Autodesk Inventor part; units mm, degrees
(part 2 of 4)
  line L580 (32.3405, 31.3602) -> (32.5714, 31.19) construction
  spline S108 degree 2 poles (32.5714, 31.19) (32.7659, 31.0482) (32.9604, 30.5985) (32.9604, 30.3229) knots 0 0 0 1 2 2 2
  line L581 (32.5714, 31.19) -> (32.7659, 31.0482) construction
  line L582 (32.7659, 31.0482) -> (32.9604, 30.5985) construction
  line L583 (32.9604, 30.5985) -> (32.9604, 30.3229) construction
  spline S109 degree 2 poles (32.9604, 30.3229) (32.9604, 30.0515) (32.7416, 29.6058) (32.5552, 29.468) knots 0 0 0 1 2 2 2
  line L584 (32.9604, 30.3229) -> (32.9604, 30.0515) construction
  line L585 (32.9604, 30.0515) -> (32.7416, 29.6058) construction
  line L586 (32.7416, 29.6058) -> (32.5552, 29.468) construction
  spline S110 degree 2 poles (35.9385, 29.5571) (35.7076, 29.7962) (35.4523, 30.5336) (35.4523, 31.028) knots 0 0 0 1 2 2 2
  line L587 (35.9385, 29.5571) -> (35.7076, 29.7962) construction
  line L588 (35.7076, 29.7962) -> (35.4523, 30.5336) construction
  line L589 (35.4523, 30.5336) -> (35.4523, 31.028) construction
  spline S111 degree 2 poles (35.4523, 31.028) (35.4523, 31.5223) (35.7157, 32.2435) (35.9385, 32.4866) knots 0 0 0 1 2 2 2
  line L590 (35.4523, 31.028) -> (35.4523, 31.5223) construction
  line L591 (35.4523, 31.5223) -> (35.7157, 32.2435) construction
  line L592 (35.7157, 32.2435) -> (35.9385, 32.4866) construction
  spline S112 degree 2 poles (35.9385, 32.4866) (36.1614, 32.7338) (36.8219, 32.9972) (37.2027, 32.9972) knots 0 0 0 1 2 2 2
  line L593 (35.9385, 32.4866) -> (36.1614, 32.7338) construction
  line L594 (36.1614, 32.7338) -> (36.8219, 32.9972) construction
  line L595 (36.8219, 32.9972) -> (37.2027, 32.9972) construction
  spline S113 degree 2 poles (37.2027, 32.9972) (37.5107, 32.9972) (38.086, 32.8229) (38.3089, 32.7095) knots 0 0 0 1 2 2 2
  line L596 (37.2027, 32.9972) -> (37.5107, 32.9972) construction
  line L597 (37.5107, 32.9972) -> (38.086, 32.8229) construction
  line L598 (38.086, 32.8229) -> (38.3089, 32.7095) construction
  spline S114 degree 2 poles (38.2724, 32.0004) (38.2035, 32.0571) (37.9928, 32.203) (37.8429, 32.28) knots 0 0 0 1 2 2 2
  line L599 (38.2724, 32.0004) -> (38.2035, 32.0571) construction
  line L600 (38.2035, 32.0571) -> (37.9928, 32.203) construction
  line L601 (37.9928, 32.203) -> (37.8429, 32.28) construction
  spline S115 degree 2 poles (37.8429, 32.28) (37.7092, 32.3448) (37.3526, 32.4461) (37.1906, 32.4461) knots 0 0 0 1 2 2 2
  line L602 (37.8429, 32.28) -> (37.7092, 32.3448) construction
  line L603 (37.7092, 32.3448) -> (37.3526, 32.4461) construction
  line L604 (37.3526, 32.4461) -> (37.1906, 32.4461) construction
  spline S116 degree 2 poles (37.1906, 32.4461) (36.7003, 32.4461) (36.1047, 31.7046) (36.1047, 31.028) knots 0 0 0 1 2 2 2
  line L605 (37.1906, 32.4461) -> (36.7003, 32.4461) construction
  line L606 (36.7003, 32.4461) -> (36.1047, 31.7046) construction
  line L607 (36.1047, 31.7046) -> (36.1047, 31.028) construction
  spline S117 degree 2 poles (36.1047, 31.028) (36.1047, 30.3675) (36.68, 29.626) (37.1906, 29.626) knots 0 0 0 1 2 2 2
  line L608 (36.1047, 31.028) -> (36.1047, 30.3675) construction
  line L609 (36.1047, 30.3675) -> (36.68, 29.626) construction
  line L610 (36.68, 29.626) -> (37.1906, 29.626) construction
  spline S118 degree 2 poles (37.1906, 29.626) (37.4985, 29.626) (38.0577, 29.8813) (38.2724, 30.0798) knots 0 0 0 1 2 2 2
  line L611 (37.1906, 29.626) -> (37.4985, 29.626) construction
  line L612 (37.4985, 29.626) -> (38.0577, 29.8813) construction
  line L613 (38.0577, 29.8813) -> (38.2724, 30.0798) construction
  spline S119 degree 2 poles (38.3089, 29.3707) (38.2157, 29.3262) (37.9321, 29.2006) (37.8186, 29.1722) knots 0 0 0 1 2 2 2
  line L614 (38.3089, 29.3707) -> (38.2157, 29.3262) construction
  line L615 (38.2157, 29.3262) -> (37.9321, 29.2006) construction
  line L616 (37.9321, 29.2006) -> (37.8186, 29.1722) construction
  spline S120 degree 2 poles (37.8186, 29.1722) (37.6565, 29.1236) (37.4013, 29.075) (37.2027, 29.075) knots 0 0 0 1 2 2 2
  line L617 (37.8186, 29.1722) -> (37.6565, 29.1236) construction
  line L618 (37.6565, 29.1236) -> (37.4013, 29.075) construction
  line L619 (37.4013, 29.075) -> (37.2027, 29.075) construction
  spline S121 degree 2 poles (37.2027, 29.075) (36.8138, 29.075) (36.1695, 29.314) (35.9385, 29.5571) knots 0 0 0 1 2 2 2
  line L620 (37.2027, 29.075) -> (36.8138, 29.075) construction
  line L621 (36.8138, 29.075) -> (36.1695, 29.314) construction
  line L622 (36.1695, 29.314) -> (35.9385, 29.5571) construction
  spline S122 degree 2 poles (36.6071, 21.7178) (36.4937, 21.4504) (36.21, 21.1303) (36.0561, 21.0492) knots 0 0 0 1 2 2 2
  line L623 (36.6071, 21.7178) -> (36.4937, 21.4504) construction
  line L624 (36.4937, 21.4504) -> (36.21, 21.1303) construction
  line L625 (36.21, 21.1303) -> (36.0561, 21.0492) construction
  spline S123 degree 2 poles (36.0561, 21.0492) (35.898, 20.9641) (35.6022, 20.9115) (35.4483, 20.9115) knots 0 0 0 1 2 2 2
  line L626 (36.0561, 21.0492) -> (35.898, 20.9641) construction
  line L627 (35.898, 20.9641) -> (35.6022, 20.9115) construction
  line L628 (35.6022, 20.9115) -> (35.4483, 20.9115) construction
  spline S124 degree 2 poles (35.4483, 20.9115) (35.3146, 20.9115) (34.9499, 20.9236) (34.9013, 20.9277) knots 0 0 0 1 2 2 2
  line L629 (35.4483, 20.9115) -> (35.3146, 20.9115) construction
  line L630 (35.3146, 20.9115) -> (34.9499, 20.9236) construction
  line L631 (34.9499, 20.9236) -> (34.9013, 20.9277) construction
  spline S125 degree 2 poles (34.9499, 21.5517) (34.9985, 21.5436) (35.2052, 21.5274) (35.3632, 21.5274) knots 0 0 0 1 2 2 2
  line L632 (34.9499, 21.5517) -> (34.9985, 21.5436) construction
  line L633 (34.9985, 21.5436) -> (35.2052, 21.5274) construction
  line L634 (35.2052, 21.5274) -> (35.3632, 21.5274) construction
  spline S126 degree 2 poles (35.3632, 21.5274) (35.4361, 21.5274) (35.6387, 21.5436) (35.7238, 21.5841) knots 0 0 0 1 2 2 2
  line L635 (35.3632, 21.5274) -> (35.4361, 21.5274) construction
  line L636 (35.4361, 21.5274) -> (35.6387, 21.5436) construction
  line L637 (35.6387, 21.5436) -> (35.7238, 21.5841) construction
  spline S127 degree 2 poles (35.7238, 21.5841) (35.821, 21.6327) (35.9912, 21.7867) (36.0601, 21.9609) knots 0 0 0 1 2 2 2
  line L638 (35.7238, 21.5841) -> (35.821, 21.6327) construction
  line L639 (35.821, 21.6327) -> (35.9912, 21.7867) construction
  line L640 (35.9912, 21.7867) -> (36.0601, 21.9609) construction
  spline S128 degree 2 poles (23.4711, -2.5288) (23.0697, -2.5288) (22.4735, -1.952) (22.4735, -1.5311) knots 0 0 0 1 2 2 2
  line L641 (23.4711, -2.5288) -> (23.0697, -2.5288) construction
  line L642 (23.0697, -2.5288) -> (22.4735, -1.952) construction
  line L643 (22.4735, -1.952) -> (22.4735, -1.5311) construction
  line L644 (22.4735, -1.5311) -> (22.4735, -0.0346)
  spline S129 degree 2 poles (22.4735, -0.0346) (22.4735, 0.3785) (23.058, 0.963) (23.4711, 0.963) knots 0 0 0 1 2 2 2
  line L645 (22.4735, -0.0346) -> (22.4735, 0.3785) construction
  line L646 (22.4735, 0.3785) -> (23.058, 0.963) construction
  line L647 (23.058, 0.963) -> (23.4711, 0.963) construction
  line L648 (23.4711, 0.963) -> (24.2194, 0.963)
  spline S130 degree 2 poles (24.2194, 0.963) (24.3207, 0.963) (24.4688, 0.8111) (24.4688, 0.7136) knots 0 0 0 1 2 2 2
  line L649 (24.2194, 0.963) -> (24.3207, 0.963) construction
  line L650 (24.3207, 0.963) -> (24.4688, 0.8111) construction
  line L651 (24.4688, 0.8111) -> (24.4688, 0.7136) construction
  spline S131 degree 2 poles (24.4688, 0.7136) (24.4688, 0.6279) (24.3441, 0.4642) (24.2194, 0.4642) knots 0 0 0 1 2 2 2
  line L652 (24.4688, 0.7136) -> (24.4688, 0.6279) construction
  line L653 (24.4688, 0.6279) -> (24.3441, 0.4642) construction
  line L654 (24.3441, 0.4642) -> (24.2194, 0.4642) construction
  line L655 (24.2194, 0.4642) -> (23.4711, 0.4642)
  spline S132 degree 2 poles (23.4711, 0.4642) (23.2607, 0.4642) (23.1165, 0.32) knots 0 0 0 1 1 1
  line L656 (23.4711, 0.4642) -> (23.2607, 0.4642) construction
  line L657 (23.2607, 0.4642) -> (23.1165, 0.32) construction
  spline S133 degree 2 poles (23.1165, 0.32) (23.0424, 0.2499) (22.9723, 0.0706) (22.9723, -0.0346) knots 0 0 0 1 2 2 2
  line L658 (23.1165, 0.32) -> (23.0424, 0.2499) construction
  line L659 (23.0424, 0.2499) -> (22.9723, 0.0706) construction
  line L660 (22.9723, 0.0706) -> (22.9723, -0.0346) construction
  line L661 (22.9723, -0.0346) -> (22.9723, -1.5311)
  spline S134 degree 2 poles (22.9723, -1.5311) (22.9723, -1.7415) (23.1165, -1.8857) knots 0 0 0 1 1 1
  line L662 (22.9723, -1.5311) -> (22.9723, -1.7415) construction
  line L663 (22.9723, -1.7415) -> (23.1165, -1.8857) construction
  spline S135 degree 2 poles (23.1165, -1.8857) (23.1905, -1.952) (23.2763, -1.9949) knots 0 0 0 1 1 1
  line L664 (23.1165, -1.8857) -> (23.1905, -1.952) construction
  line L665 (23.1905, -1.952) -> (23.2763, -1.9949) construction
  spline S136 degree 2 poles (23.2763, -1.9949) (23.3815, -2.0299) (23.4711, -2.0299) knots 0 0 0 1 1 1
  line L666 (23.2763, -1.9949) -> (23.3815, -2.0299) construction
  line L667 (23.3815, -2.0299) -> (23.4711, -2.0299) construction
  line L668 (23.4711, -2.0299) -> (24.2194, -2.0299)
  spline S137 degree 2 poles (24.2194, -2.0299) (24.3207, -2.0299) (24.4688, -2.1819) (24.4688, -2.2794) knots 0 0 0 1 2 2 2
  line L669 (24.2194, -2.0299) -> (24.3207, -2.0299) construction
  line L670 (24.3207, -2.0299) -> (24.4688, -2.1819) construction
  line L671 (24.4688, -2.1819) -> (24.4688, -2.2794) construction
  spline S138 degree 2 poles (24.4688, -2.2794) (24.4688, -2.3651) (24.3441, -2.5288) (24.2194, -2.5288) knots 0 0 0 1 2 2 2
  line L672 (24.4688, -2.2794) -> (24.4688, -2.3651) construction
  line L673 (24.4688, -2.3651) -> (24.3441, -2.5288) construction
  line L674 (24.3441, -2.5288) -> (24.2194, -2.5288) construction
  line L675 (24.2194, -2.5288) -> (23.4711, -2.5288)
  spline S139 degree 2 poles (2.1309, -41.5414) (1.6445, -41.5414) (0.9337, -40.8446) (0.9337, -40.3442) knots 0 0 0 1 2 2 2
  line L676 (2.1309, -41.5414) -> (1.6445, -41.5414) construction
  line L677 (1.6445, -41.5414) -> (0.9337, -40.8446) construction
  line L678 (0.9337, -40.8446) -> (0.9337, -40.3442) construction
  line L679 (0.9337, -40.3442) -> (0.9337, -36.7526)
  spline S140 degree 2 poles (0.9337, -36.7526) (0.9337, -36.2522) (1.6305, -35.5554) (2.1309, -35.5554) knots 0 0 0 1 2 2 2
  line L680 (0.9337, -36.7526) -> (0.9337, -36.2522) construction
  line L681 (0.9337, -36.2522) -> (1.6305, -35.5554) construction
  line L682 (1.6305, -35.5554) -> (2.1309, -35.5554) construction
  line L683 (2.1309, -35.5554) -> (3.6274, -35.5554)
  spline S141 degree 2 poles (3.6274, -35.5554) (3.749, -35.5554) (3.9267, -35.7378) (3.9267, -35.8547) knots 0 0 0 1 2 2 2
  line L684 (3.6274, -35.5554) -> (3.749, -35.5554) construction
  line L685 (3.749, -35.5554) -> (3.9267, -35.7378) construction
  line L686 (3.9267, -35.7378) -> (3.9267, -35.8547) construction
  spline S142 degree 2 poles (3.9267, -35.8547) (3.9267, -35.9576) (3.777, -36.154) (3.6274, -36.154) knots 0 0 0 1 2 2 2
  line L687 (3.9267, -35.8547) -> (3.9267, -35.9576) construction
  line L688 (3.9267, -35.9576) -> (3.777, -36.154) construction
  line L689 (3.777, -36.154) -> (3.6274, -36.154) construction
  line L690 (3.6274, -36.154) -> (2.1309, -36.154)
  spline S143 degree 2 poles (2.1309, -36.154) (1.8784, -36.154) (1.7053, -36.3271) knots 0 0 0 1 1 1
  line L691 (2.1309, -36.154) -> (1.8784, -36.154) construction
  line L692 (1.8784, -36.154) -> (1.7053, -36.3271) construction
  spline S144 degree 2 poles (1.7053, -36.3271) (1.6165, -36.4112) (1.5323, -36.6263) (1.5323, -36.7526) knots 0 0 0 1 2 2 2
  line L693 (1.7053, -36.3271) -> (1.6165, -36.4112) construction
  line L694 (1.6165, -36.4112) -> (1.5323, -36.6263) construction
  line L695 (1.5323, -36.6263) -> (1.5323, -36.7526) construction
  line L696 (1.5323, -36.7526) -> (1.5323, -40.3442)
  spline S145 degree 2 poles (1.5323, -40.3442) (1.5323, -40.5967) (1.7053, -40.7698) knots 0 0 0 1 1 1
  line L697 (1.5323, -40.3442) -> (1.5323, -40.5967) construction
  line L698 (1.5323, -40.5967) -> (1.7053, -40.7698) construction
  spline S146 degree 2 poles (1.7053, -40.7698) (1.7942, -40.8493) (1.8971, -40.9007) knots 0 0 0 1 1 1
  line L699 (1.7053, -40.7698) -> (1.7942, -40.8493) construction
  line L700 (1.7942, -40.8493) -> (1.8971, -40.9007) construction
  spline S147 degree 2 poles (1.8971, -40.9007) (2.0233, -40.9428) (2.1309, -40.9428) knots 0 0 0 1 1 1
  line L701 (1.8971, -40.9007) -> (2.0233, -40.9428) construction
  line L702 (2.0233, -40.9428) -> (2.1309, -40.9428) construction
  line L703 (2.1309, -40.9428) -> (3.6274, -40.9428)
  spline S148 degree 2 poles (3.6274, -40.9428) (3.749, -40.9428) (3.9267, -41.1252) (3.9267, -41.2421) knots 0 0 0 1 2 2 2
  line L704 (3.6274, -40.9428) -> (3.749, -40.9428) construction
  line L705 (3.749, -40.9428) -> (3.9267, -41.1252) construction
  line L706 (3.9267, -41.1252) -> (3.9267, -41.2421) construction
  spline S149 degree 2 poles (3.9267, -41.2421) (3.9267, -41.345) (3.777, -41.5414) (3.6274, -41.5414) knots 0 0 0 1 2 2 2
  line L707 (3.9267, -41.2421) -> (3.9267, -41.345) construction
  line L708 (3.9267, -41.345) -> (3.777, -41.5414) construction
  line L709 (3.777, -41.5414) -> (3.6274, -41.5414) construction
  line L710 (3.6274, -41.5414) -> (2.1309, -41.5414)
  spline S150 degree 2 poles (-5.1364, -41.4666) (-5.2206, -41.5414) (-5.3516, -41.5414) knots 0 0 0 1 1 1
  line L711 (-5.1364, -41.4666) -> (-5.2206, -41.5414) construction
  line L712 (-5.2206, -41.5414) -> (-5.3516, -41.5414) construction
  spline S151 degree 2 poles (-5.3516, -41.5414) (-5.4732, -41.5414) (-5.6509, -41.3917) (-5.6509, -41.2421) knots 0 0 0 1 2 2 2
  line L713 (-5.3516, -41.5414) -> (-5.4732, -41.5414) construction
  line L714 (-5.4732, -41.5414) -> (-5.6509, -41.3917) construction
  line L715 (-5.6509, -41.3917) -> (-5.6509, -41.2421) construction
  spline S152 degree 2 poles (-8.0452, -41.2421) (-8.0452, -41.3824) (-8.1294, -41.4666) knots 0 0 0 1 1 1
  line L716 (-8.0452, -41.2421) -> (-8.0452, -41.3824) construction
  line L717 (-8.0452, -41.3824) -> (-8.1294, -41.4666) construction
  spline S153 degree 2 poles (-8.1294, -41.4666) (-8.2136, -41.5414) (-8.3445, -41.5414) knots 0 0 0 1 1 1
  line L718 (-8.1294, -41.4666) -> (-8.2136, -41.5414) construction
  line L719 (-8.2136, -41.5414) -> (-8.3445, -41.5414) construction
  spline S154 degree 2 poles (-8.3445, -41.5414) (-8.4661, -41.5414) (-8.6438, -41.3917) (-8.6438, -41.2421) knots 0 0 0 1 2 2 2
  line L720 (-8.3445, -41.5414) -> (-8.4661, -41.5414) construction
  line L721 (-8.4661, -41.5414) -> (-8.6438, -41.3917) construction
  line L722 (-8.6438, -41.3917) -> (-8.6438, -41.2421) construction
  line L723 (-8.6438, -41.2421) -> (-8.6438, -35.8547)
  spline S155 degree 2 poles (-8.6438, -35.8547) (-8.6438, -35.5554) (-8.3445, -35.5554) knots 0 0 0 1 1 1
  line L724 (-8.6438, -35.8547) -> (-8.6438, -35.5554) construction
  line L725 (-8.6438, -35.5554) -> (-8.3445, -35.5554) construction
  line L726 (-8.3445, -35.5554) -> (-5.3516, -35.5554)
  spline S156 degree 2 poles (-5.3516, -35.5554) (-5.0523, -35.5554) (-5.0523, -35.8547) knots 0 0 0 1 1 1
  line L727 (-5.3516, -35.5554) -> (-5.0523, -35.5554) construction
  line L728 (-5.0523, -35.5554) -> (-5.0523, -35.8547) construction
  line L729 (-5.0523, -35.8547) -> (-5.0523, -41.2421)
  spline S157 degree 2 poles (-5.0523, -41.2421) (-5.0523, -41.3824) (-5.1364, -41.4666) knots 0 0 0 1 1 1
  line L730 (-5.0523, -41.2421) -> (-5.0523, -41.3824) construction
  line L731 (-5.0523, -41.3824) -> (-5.1364, -41.4666) construction
  spline S158 degree 2 poles (-28.9828, -2.8867) (-29.3881, -2.8867) (-29.9804, -2.306) (-29.9804, -1.889) knots 0 0 0 1 2 2 2
  line L732 (-28.9828, -2.8867) -> (-29.3881, -2.8867) construction
  line L733 (-29.3881, -2.8867) -> (-29.9804, -2.306) construction
  line L734 (-29.9804, -2.306) -> (-29.9804, -1.889) construction
  line L735 (-29.9804, -1.889) -> (-29.9804, 1.104)
  spline S159 degree 2 poles (-29.9804, 1.104) (-29.9804, 1.5209) (-29.3998, 2.1016) (-28.9828, 2.1016) knots 0 0 0 1 2 2 2
  line L736 (-29.9804, 1.104) -> (-29.9804, 1.5209) construction
  line L737 (-29.9804, 1.5209) -> (-29.3998, 2.1016) construction
  line L738 (-29.3998, 2.1016) -> (-28.9828, 2.1016) construction
  line L739 (-28.9828, 2.1016) -> (-27.7357, 2.1016)
  spline S160 degree 2 poles (-27.7357, 2.1016) (-27.6344, 2.1016) (-27.4863, 1.9496) (-27.4863, 1.8522) knots 0 0 0 1 2 2 2
  line L740 (-27.7357, 2.1016) -> (-27.6344, 2.1016) construction
  line L741 (-27.6344, 2.1016) -> (-27.4863, 1.9496) construction
  line L742 (-27.4863, 1.9496) -> (-27.4863, 1.8522) construction
  spline S161 degree 2 poles (-27.4863, 1.8522) (-27.4863, 1.7665) (-27.611, 1.6028) (-27.7357, 1.6028) knots 0 0 0 1 2 2 2
  line L743 (-27.4863, 1.8522) -> (-27.4863, 1.7665) construction
  line L744 (-27.4863, 1.7665) -> (-27.611, 1.6028) construction
  line L745 (-27.611, 1.6028) -> (-27.7357, 1.6028) construction
  line L746 (-27.7357, 1.6028) -> (-28.9828, 1.6028)
  spline S162 degree 2 poles (-28.9828, 1.6028) (-29.1932, 1.6028) (-29.3374, 1.4586) knots 0 0 0 1 1 1
  line L747 (-28.9828, 1.6028) -> (-29.1932, 1.6028) construction
  line L748 (-29.1932, 1.6028) -> (-29.3374, 1.4586) construction
  spline S163 degree 2 poles (-29.3374, 1.4586) (-29.4114, 1.3884) (-29.4816, 1.2092) (-29.4816, 1.104) knots 0 0 0 1 2 2 2
  line L749 (-29.3374, 1.4586) -> (-29.4114, 1.3884) construction
  line L750 (-29.4114, 1.3884) -> (-29.4816, 1.2092) construction
  line L751 (-29.4816, 1.2092) -> (-29.4816, 1.104) construction
  line L752 (-29.4816, 1.104) -> (-29.4816, -1.889)
  spline S164 degree 2 poles (-29.4816, -1.889) (-29.4816, -2.0995) (-29.3374, -2.2437) knots 0 0 0 1 1 1
  line L753 (-29.4816, -1.889) -> (-29.4816, -2.0995) construction
  line L754 (-29.4816, -2.0995) -> (-29.3374, -2.2437) construction
  spline S165 degree 2 poles (-29.3374, -2.2437) (-29.2634, -2.3099) (-29.1776, -2.3528) knots 0 0 0 1 1 1
  line L755 (-29.3374, -2.2437) -> (-29.2634, -2.3099) construction
  line L756 (-29.2634, -2.3099) -> (-29.1776, -2.3528) construction
  spline S166 degree 2 poles (-29.1776, -2.3528) (-29.0724, -2.3879) (-28.9828, -2.3879) knots 0 0 0 1 1 1
  line L757 (-29.1776, -2.3528) -> (-29.0724, -2.3879) construction
  line L758 (-29.0724, -2.3879) -> (-28.9828, -2.3879) construction
  line L759 (-28.9828, -2.3879) -> (-27.7357, -2.3879)
  spline S167 degree 2 poles (-27.7357, -2.3879) (-27.6344, -2.3879) (-27.4863, -2.5398) (-27.4863, -2.6373) knots 0 0 0 1 2 2 2
  line L760 (-27.7357, -2.3879) -> (-27.6344, -2.3879) construction
  line L761 (-27.6344, -2.3879) -> (-27.4863, -2.5398) construction
  line L762 (-27.4863, -2.5398) -> (-27.4863, -2.6373) construction
  spline S168 degree 2 poles (-27.4863, -2.6373) (-27.4863, -2.723) (-27.611, -2.8867) (-27.7357, -2.8867) knots 0 0 0 1 2 2 2
  line L763 (-27.4863, -2.6373) -> (-27.4863, -2.723) construction
  line L764 (-27.4863, -2.723) -> (-27.611, -2.8867) construction
  line L765 (-27.611, -2.8867) -> (-27.7357, -2.8867) construction
  line L766 (-27.7357, -2.8867) -> (-28.9828, -2.8867)
  spline S169 degree 2 poles (-36.2158, -0.3964) (-36.3288, -0.3964) (-36.4029, -0.3263) knots 0 0 0 1 1 1
  line L767 (-36.2158, -0.3964) -> (-36.3288, -0.3964) construction
  line L768 (-36.3288, -0.3964) -> (-36.4029, -0.3263) construction
  spline S170 degree 2 poles (-36.4029, -0.3263) (-36.4652, -0.2522) (-36.4652, -0.147) knots 0 0 0 1 1 1
  line L769 (-36.4029, -0.3263) -> (-36.4652, -0.2522) construction
  line L770 (-36.4652, -0.2522) -> (-36.4652, -0.147) construction
  spline S171 degree 2 poles (-36.4652, -0.147) (-36.4652, -0.0574) (-36.3327, 0.1024) (-36.2158, 0.1024) knots 0 0 0 1 2 2 2
  line L771 (-36.4652, -0.147) -> (-36.4652, -0.0574) construction
  line L772 (-36.4652, -0.0574) -> (-36.3327, 0.1024) construction
  line L773 (-36.3327, 0.1024) -> (-36.2158, 0.1024) construction
  spline S172 degree 2 poles (-34.9687, 1.104) (-34.9687, 1.3144) (-35.2493, 1.6028) (-35.4676, 1.6028) knots 0 0 0 1 2 2 2
  line L774 (-34.9687, 1.104) -> (-34.9687, 1.3144) construction
  line L775 (-34.9687, 1.3144) -> (-35.2493, 1.6028) construction
  line L776 (-35.2493, 1.6028) -> (-35.4676, 1.6028) construction
  line L777 (-35.4676, 1.6028) -> (-37.2135, 1.6028)
  spline S173 degree 2 poles (-37.2135, 1.6028) (-37.3265, 1.6028) (-37.4005, 1.669) knots 0 0 0 1 1 1
  line L778 (-37.2135, 1.6028) -> (-37.3265, 1.6028) construction
  line L779 (-37.3265, 1.6028) -> (-37.4005, 1.669) construction
  spline S174 degree 2 poles (-37.4005, 1.669) (-37.4629, 1.7509) (-37.4629, 1.8522) knots 0 0 0 1 1 1
  line L780 (-37.4005, 1.669) -> (-37.4629, 1.7509) construction
  line L781 (-37.4629, 1.7509) -> (-37.4629, 1.8522) construction
  spline S175 degree 2 poles (-37.4629, 1.8522) (-37.4629, 1.9379) (-37.3382, 2.1016) (-37.2135, 2.1016) knots 0 0 0 1 2 2 2
  line L782 (-37.4629, 1.8522) -> (-37.4629, 1.9379) construction
  line L783 (-37.4629, 1.9379) -> (-37.3382, 2.1016) construction
  line L784 (-37.3382, 2.1016) -> (-37.2135, 2.1016) construction
  line L785 (-37.2135, 2.1016) -> (-35.4676, 2.1016)
  spline S176 degree 2 poles (-35.4676, 2.1016) (-35.0506, 2.1016) (-34.4699, 1.517) (-34.4699, 1.104) knots 0 0 0 1 2 2 2
  line L786 (-35.4676, 2.1016) -> (-35.0506, 2.1016) construction
  line L787 (-35.0506, 2.1016) -> (-34.4699, 1.517) construction
  line L788 (-34.4699, 1.517) -> (-34.4699, 1.104) construction
  line L789 (-34.4699, 1.104) -> (-34.4699, -1.889)
  spline S177 degree 2 poles (-34.4699, -1.889) (-34.4699, -2.2982) (-35.0545, -2.8867) (-35.4676, -2.8867) knots 0 0 0 1 2 2 2
  line L790 (-34.4699, -1.889) -> (-34.4699, -2.2982) construction
  line L791 (-34.4699, -2.2982) -> (-35.0545, -2.8867) construction
  line L792 (-35.0545, -2.8867) -> (-35.4676, -2.8867) construction
  line L793 (-35.4676, -2.8867) -> (-37.2135, -2.8867)
  spline S178 degree 2 poles (-37.2135, -2.8867) (-37.3265, -2.8867) (-37.4005, -2.8165) knots 0 0 0 1 1 1
  line L794 (-37.2135, -2.8867) -> (-37.3265, -2.8867) construction
  line L795 (-37.3265, -2.8867) -> (-37.4005, -2.8165) construction
  spline S179 degree 2 poles (-37.4005, -2.8165) (-37.4629, -2.7425) (-37.4629, -2.6373) knots 0 0 0 1 1 1
  line L796 (-37.4005, -2.8165) -> (-37.4629, -2.7425) construction
  line L797 (-37.4629, -2.7425) -> (-37.4629, -2.6373) construction
  spline S180 degree 2 poles (-37.4629, -2.6373) (-37.4629, -2.5476) (-37.3304, -2.3879) (-37.2135, -2.3879) knots 0 0 0 1 2 2 2
  line L798 (-37.4629, -2.6373) -> (-37.4629, -2.5476) construction
  line L799 (-37.4629, -2.5476) -> (-37.3304, -2.3879) construction
  line L800 (-37.3304, -2.3879) -> (-37.2135, -2.3879) construction
  line L801 (-37.2135, -2.3879) -> (-35.4676, -2.3879)
  spline S181 degree 2 poles (-35.4676, -2.3879) (-35.261, -2.3879) (-34.9687, -2.1112) (-34.9687, -1.889) knots 0 0 0 1 2 2 2
  line L802 (-35.4676, -2.3879) -> (-35.261, -2.3879) construction
  line L803 (-35.261, -2.3879) -> (-34.9687, -2.1112) construction
  line L804 (-34.9687, -2.1112) -> (-34.9687, -1.889) construction
  spline S182 degree 2 poles (-26.032, -101.232) (-25.6557, -101.232) (-25.4359, -101.4818) knots 0 0 0 1 1 1
  line L805 (-26.032, -101.232) -> (-25.6557, -101.232) construction
  line L806 (-25.6557, -101.232) -> (-25.4359, -101.4818) construction
  spline S183 degree 2 poles (-25.4359, -101.4818) (-25.236, -101.705) (-25.236, -102.0281) knots 0 0 0 1 1 1
  line L807 (-25.4359, -101.4818) -> (-25.236, -101.705) construction
  line L808 (-25.236, -101.705) -> (-25.236, -102.0281) construction
  spline S184 degree 2 poles (-25.236, -102.0281) (-25.236, -102.3511) (-25.4359, -102.5809) knots 0 0 0 1 1 1
  line L809 (-25.236, -102.0281) -> (-25.236, -102.3511) construction
  line L810 (-25.236, -102.3511) -> (-25.4359, -102.5809) construction
  spline S185 degree 2 poles (-25.4359, -102.5809) (-25.6557, -102.8274) (-26.032, -102.8274) knots 0 0 0 1 1 1
  line L811 (-25.4359, -102.5809) -> (-25.6557, -102.8274) construction
  line L812 (-25.6557, -102.8274) -> (-26.032, -102.8274) construction
  line L813 (-26.032, -102.8274) -> (-26.6315, -102.8274)
  spline S186 degree 2 poles (-26.6315, -102.8274) (-26.8314, -102.8274) (-26.8314, -102.6276) knots 0 0 0 1 1 1
  line L814 (-26.6315, -102.8274) -> (-26.8314, -102.8274) construction
  line L815 (-26.8314, -102.8274) -> (-26.8314, -102.6276) construction
  line L816 (-26.8314, -102.6276) -> (-26.8314, -100.2362)
  spline S187 degree 2 poles (-26.8314, -100.2362) (-26.8314, -100.0364) (-26.6315, -100.0364) knots 0 0 0 1 1 1
  line L817 (-26.8314, -100.2362) -> (-26.8314, -100.0364) construction
  line L818 (-26.8314, -100.0364) -> (-26.6315, -100.0364) construction
  spline S188 degree 2 poles (-26.6315, -100.0364) (-26.4317, -100.0364) (-26.4317, -100.2362) knots 0 0 0 1 1 1
  line L819 (-26.6315, -100.0364) -> (-26.4317, -100.0364) construction
  line L820 (-26.4317, -100.0364) -> (-26.4317, -100.2362) construction
  spline S189 degree 2 poles (-29.2227, -103.8232) (-29.2227, -104.0231) (-29.4225, -104.0231) knots 0 0 0 1 1 1
  line L821 (-29.2227, -103.8232) -> (-29.2227, -104.0231) construction
  line L822 (-29.2227, -104.0231) -> (-29.4225, -104.0231) construction
  spline S190 degree 2 poles (-29.4225, -104.0231) (-29.6224, -104.0231) (-29.6224, -103.8232) knots 0 0 0 1 1 1
  line L823 (-29.4225, -104.0231) -> (-29.6224, -104.0231) construction
  line L824 (-29.6224, -104.0231) -> (-29.6224, -103.8232) construction
  line L825 (-29.6224, -103.8232) -> (-29.6224, -100.2362)
  spline S191 degree 2 poles (-29.6224, -100.2362) (-29.6224, -100.0364) (-29.4225, -100.0364) knots 0 0 0 1 1 1
  line L826 (-29.6224, -100.2362) -> (-29.6224, -100.0364) construction
  line L827 (-29.6224, -100.0364) -> (-29.4225, -100.0364) construction
  line L828 (-29.4225, -100.0364) -> (-28.4267, -100.0364)
  spline S192 degree 2 poles (-28.4267, -100.0364) (-28.097, -100.0364) (-27.6307, -100.5027) (-27.6307, -100.8324) knots 0 0 0 1 2 2 2
  line L829 (-28.4267, -100.0364) -> (-28.097, -100.0364) construction
  line L830 (-28.097, -100.0364) -> (-27.6307, -100.5027) construction
  line L831 (-27.6307, -100.5027) -> (-27.6307, -100.8324) construction
  line L832 (-27.6307, -100.8324) -> (-27.6307, -102.0314)
  spline S193 degree 2 poles (-27.6307, -102.0314) (-27.6307, -102.3611) (-28.097, -102.8274) (-28.4267, -102.8274) knots 0 0 0 1 2 2 2
  line L833 (-27.6307, -102.0314) -> (-27.6307, -102.3611) construction
  line L834 (-27.6307, -102.3611) -> (-28.097, -102.8274) construction
  line L835 (-28.097, -102.8274) -> (-28.4267, -102.8274) construction
  spline S194 degree 2 poles (3.5401, 27.5031) (3.5401, 27.3862) (3.4699, 27.316) knots 0 0 0 1 1 1
  line L836 (3.5401, 27.5031) -> (3.5401, 27.3862) construction
  line L837 (3.5401, 27.3862) -> (3.4699, 27.316) construction
  spline S195 degree 2 poles (3.4699, 27.316) (3.3998, 27.2537) (3.2907, 27.2537) knots 0 0 0 1 1 1
  line L838 (3.4699, 27.316) -> (3.3998, 27.2537) construction
  line L839 (3.3998, 27.2537) -> (3.2907, 27.2537) construction
  spline S196 degree 2 poles (3.2907, 27.2537) (3.1893, 27.2537) (3.0412, 27.3784) (3.0412, 27.5031) knots 0 0 0 1 2 2 2
  line L840 (3.2907, 27.2537) -> (3.1893, 27.2537) construction
  line L841 (3.1893, 27.2537) -> (3.0412, 27.3784) construction
  line L842 (3.0412, 27.3784) -> (3.0412, 27.5031) construction
  line L843 (3.0412, 27.5031) -> (3.0412, 30.4961)
  spline S197 degree 2 poles (3.0412, 30.4961) (3.0412, 30.5935) (3.1153, 30.6793) knots 0 0 0 1 1 1
  line L844 (3.0412, 30.4961) -> (3.0412, 30.5935) construction
  line L845 (3.0412, 30.5935) -> (3.1153, 30.6793) construction
  spline S198 degree 2 poles (3.1153, 30.6793) (3.1893, 30.7455) (3.2907, 30.7455) knots 0 0 0 1 1 1
  line L846 (3.1153, 30.6793) -> (3.1893, 30.7455) construction
  line L847 (3.1893, 30.7455) -> (3.2907, 30.7455) construction
  spline S199 degree 2 poles (3.2907, 30.7455) (3.3881, 30.7455) (3.5401, 30.6208) (3.5401, 30.4961) knots 0 0 0 1 2 2 2
  line L848 (3.2907, 30.7455) -> (3.3881, 30.7455) construction
  line L849 (3.3881, 30.7455) -> (3.5401, 30.6208) construction
  line L850 (3.5401, 30.6208) -> (3.5401, 30.4961) construction
  spline S200 degree 2 poles (5.1223, 30.6831) (5.1847, 30.7572) (5.2821, 30.7572) knots 0 0 0 1 1 1
  line L851 (5.1223, 30.6831) -> (5.1847, 30.7572) construction
  line L852 (5.1847, 30.7572) -> (5.2821, 30.7572) construction
  spline S201 degree 2 poles (5.2821, 30.7572) (5.36, 30.7572) (5.4574, 30.6831) knots 0 0 0 1 1 1
  line L853 (5.2821, 30.7572) -> (5.36, 30.7572) construction
  line L854 (5.36, 30.7572) -> (5.4574, 30.6831) construction
  spline S202 degree 2 poles (5.4574, 30.6831) (5.5315, 30.6091) (5.5315, 30.4922) knots 0 0 0 1 1 1
  line L855 (5.4574, 30.6831) -> (5.5315, 30.6091) construction
  line L856 (5.5315, 30.6091) -> (5.5315, 30.4922) construction
  spline S203 degree 2 poles (5.5315, 30.4922) (5.5315, 30.3909) (5.4497, 30.3051) knots 0 0 0 1 1 1
  line L857 (5.5315, 30.4922) -> (5.5315, 30.3909) construction
  line L858 (5.5315, 30.3909) -> (5.4497, 30.3051) construction
  spline S204 degree 2 poles (5.473, 27.6629) (5.5315, 27.5577) (5.5315, 27.4914) knots 0 0 0 1 1 1
  line L859 (5.473, 27.6629) -> (5.5315, 27.5577) construction
  line L860 (5.5315, 27.5577) -> (5.5315, 27.4914) construction
  spline S205 degree 2 poles (5.5315, 27.4914) (5.5315, 27.3862) (5.4497, 27.316) knots 0 0 0 1 1 1
  line L861 (5.5315, 27.4914) -> (5.5315, 27.3862) construction
  line L862 (5.5315, 27.3862) -> (5.4497, 27.316) construction
  spline S206 degree 2 poles (5.4497, 27.316) (5.3756, 27.242) (5.2743, 27.242) knots 0 0 0 1 1 1
  line L863 (5.4497, 27.316) -> (5.3756, 27.242) construction
  line L864 (5.3756, 27.242) -> (5.2743, 27.242) construction
  spline S207 degree 2 poles (5.2743, 27.242) (5.1769, 27.242) (5.095, 27.3433) knots 0 0 0 1 1 1
  line L865 (5.2743, 27.242) -> (5.1769, 27.242) construction
  line L866 (5.1769, 27.242) -> (5.095, 27.3433) construction
  spline S208 degree 2 poles (-2.3952, 27.2537) (-2.7966, 27.2537) (-3.3929, 27.8305) (-3.3929, 28.2513) knots 0 0 0 1 2 2 2
  line L867 (-2.3952, 27.2537) -> (-2.7966, 27.2537) construction
  line L868 (-2.7966, 27.2537) -> (-3.3929, 27.8305) construction
  line L869 (-3.3929, 27.8305) -> (-3.3929, 28.2513) construction
  line L870 (-3.3929, 28.2513) -> (-3.3929, 30.4961)
  spline S209 degree 2 poles (-3.3929, 30.4961) (-3.3929, 30.5974) (-3.3189, 30.6831) knots 0 0 0 1 1 1
  line L871 (-3.3929, 30.4961) -> (-3.3929, 30.5974) construction
  line L872 (-3.3929, 30.5974) -> (-3.3189, 30.6831) construction
  spline S210 degree 2 poles (-3.3189, 30.6831) (-3.2448, 30.7455) (-3.1435, 30.7455) knots 0 0 0 1 1 1
  line L873 (-3.3189, 30.6831) -> (-3.2448, 30.7455) construction
  line L874 (-3.2448, 30.7455) -> (-3.1435, 30.7455) construction
  spline S211 degree 2 poles (-3.1435, 30.7455) (-3.0461, 30.7455) (-2.8941, 30.6208) (-2.8941, 30.4961) knots 0 0 0 1 2 2 2
  line L875 (-3.1435, 30.7455) -> (-3.0461, 30.7455) construction
  line L876 (-3.0461, 30.7455) -> (-2.8941, 30.6208) construction
  line L877 (-2.8941, 30.6208) -> (-2.8941, 30.4961) construction
  line L878 (-2.8941, 30.4961) -> (-2.8941, 28.2513)
  spline S212 degree 2 poles (-2.8941, 28.2513) (-2.8941, 28.0409) (-2.7499, 27.8967) knots 0 0 0 1 1 1
  line L879 (-2.8941, 28.2513) -> (-2.8941, 28.0409) construction
  line L880 (-2.8941, 28.0409) -> (-2.7499, 27.8967) construction
  spline S213 degree 2 poles (-2.7499, 27.8967) (-2.6758, 27.8305) (-2.5901, 27.7876) knots 0 0 0 1 1 1
  line L881 (-2.7499, 27.8967) -> (-2.6758, 27.8305) construction
  line L882 (-2.6758, 27.8305) -> (-2.5901, 27.7876) construction
  spline S214 degree 2 poles (-2.5901, 27.7876) (-2.4849, 27.7525) (-2.3952, 27.7525) knots 0 0 0 1 1 1
  line L883 (-2.5901, 27.7876) -> (-2.4849, 27.7525) construction
  line L884 (-2.4849, 27.7525) -> (-2.3952, 27.7525) construction
  spline S215 degree 2 poles (-1.3976, 30.4961) (-1.3976, 30.5974) (-1.3235, 30.6831) knots 0 0 0 1 1 1
  line L885 (-1.3976, 30.4961) -> (-1.3976, 30.5974) construction
  line L886 (-1.3976, 30.5974) -> (-1.3235, 30.6831) construction
  spline S216 degree 2 poles (-1.3235, 30.6831) (-1.2495, 30.7455) (-1.1482, 30.7455) knots 0 0 0 1 1 1
  line L887 (-1.3235, 30.6831) -> (-1.2495, 30.7455) construction
  line L888 (-1.2495, 30.7455) -> (-1.1482, 30.7455) construction
  spline S217 degree 2 poles (-1.1482, 30.7455) (-1.0507, 30.7455) (-0.8987, 30.6208) (-0.8987, 30.4961) knots 0 0 0 1 2 2 2
  line L889 (-1.1482, 30.7455) -> (-1.0507, 30.7455) construction
  line L890 (-1.0507, 30.7455) -> (-0.8987, 30.6208) construction
  line L891 (-0.8987, 30.6208) -> (-0.8987, 30.4961) construction
  line L892 (-0.8987, 30.4961) -> (-0.8987, 26.7549)
  spline S218 degree 2 poles (-0.8987, 26.7549) (-0.8987, 26.3496) (-1.4794, 25.7572) (-1.8964, 25.7572) knots 0 0 0 1 2 2 2
  line L893 (-0.8987, 26.7549) -> (-0.8987, 26.3496) construction
  line L894 (-0.8987, 26.3496) -> (-1.4794, 25.7572) construction
  line L895 (-1.4794, 25.7572) -> (-1.8964, 25.7572) construction
  line L896 (-1.8964, 25.7572) -> (-2.8941, 25.7572)
  spline S219 degree 2 poles (-2.8941, 25.7572) (-2.9876, 25.7572) (-3.0811, 25.8312) knots 0 0 0 1 1 1
  line L897 (-2.8941, 25.7572) -> (-2.9876, 25.7572) construction
  line L898 (-2.9876, 25.7572) -> (-3.0811, 25.8312) construction
  spline S220 degree 2 poles (-3.0811, 25.8312) (-3.1435, 25.9053) (-3.1435, 26.0066) knots 0 0 0 1 1 1
  line L899 (-3.0811, 25.8312) -> (-3.1435, 25.9053) construction
  line L900 (-3.1435, 25.9053) -> (-3.1435, 26.0066) construction
  spline S221 degree 2 poles (-3.1435, 26.0066) (-3.1435, 26.1079) (-3.0188, 26.256) (-2.8941, 26.256) knots 0 0 0 1 2 2 2
  line L901 (-3.1435, 26.0066) -> (-3.1435, 26.1079) construction
  line L902 (-3.1435, 26.1079) -> (-3.0188, 26.256) construction
  line L903 (-3.0188, 26.256) -> (-2.8941, 26.256) construction
  line L904 (-2.8941, 26.256) -> (-1.8964, 26.256)
  spline S222 degree 2 poles (-1.8964, 26.256) (-1.686, 26.256) (-1.3976, 26.5366) (-1.3976, 26.7549) knots 0 0 0 1 2 2 2
  line L905 (-1.8964, 26.256) -> (-1.686, 26.256) construction
  line L906 (-1.686, 26.256) -> (-1.3976, 26.5366) construction
  line L907 (-1.3976, 26.5366) -> (-1.3976, 26.7549) construction
  spline S223 degree 2 poles (7.8308, 34.5821) (7.8308, 34.6834) (7.9048, 34.7692) knots 0 0 0 1 1 1
  line L908 (7.8308, 34.5821) -> (7.8308, 34.6834) construction
  line L909 (7.8308, 34.6834) -> (7.9048, 34.7692) construction
  spline S224 degree 2 poles (7.9048, 34.7692) (7.9789, 34.8315) (8.0802, 34.8315) knots 0 0 0 1 1 1
  line L910 (7.9048, 34.7692) -> (7.9789, 34.8315) construction
  line L911 (7.9789, 34.8315) -> (8.0802, 34.8315) construction
  spline S225 degree 2 poles (8.0802, 34.8315) (8.1776, 34.8315) (8.3296, 34.7068) (8.3296, 34.5821) knots 0 0 0 1 2 2 2
  line L912 (8.0802, 34.8315) -> (8.1776, 34.8315) construction
  line L913 (8.1776, 34.8315) -> (8.3296, 34.7068) construction
  line L914 (8.3296, 34.7068) -> (8.3296, 34.5821) construction
  line L915 (8.3296, 34.5821) -> (8.3296, 31.5891)
  spline S226 degree 2 poles (8.3296, 31.5891) (8.3296, 31.4722) (8.2595, 31.4021) knots 0 0 0 1 1 1
  line L916 (8.3296, 31.5891) -> (8.3296, 31.4722) construction
  line L917 (8.3296, 31.4722) -> (8.2595, 31.4021) construction
  spline S227 degree 2 poles (8.2595, 31.4021) (8.1893, 31.3397) (8.0802, 31.3397) knots 0 0 0 1 1 1
  line L918 (8.2595, 31.4021) -> (8.1893, 31.3397) construction
  line L919 (8.1893, 31.3397) -> (8.0802, 31.3397) construction
  spline S228 degree 2 poles (8.0802, 31.3397) (7.9789, 31.3397) (7.8308, 31.4644) (7.8308, 31.5891) knots 0 0 0 1 2 2 2
  line L920 (8.0802, 31.3397) -> (7.9789, 31.3397) construction
  line L921 (7.9789, 31.3397) -> (7.8308, 31.4644) construction
  line L922 (7.8308, 31.4644) -> (7.8308, 31.5891) construction
  spline S229 degree 2 poles (6.3343, 31.5891) (6.3343, 31.4722) (6.2642, 31.4021) knots 0 0 0 1 1 1
  line L923 (6.3343, 31.5891) -> (6.3343, 31.4722) construction
  line L924 (6.3343, 31.4722) -> (6.2642, 31.4021) construction
  spline S230 degree 2 poles (6.2642, 31.4021) (6.194, 31.3397) (6.0849, 31.3397) knots 0 0 0 1 1 1
  line L925 (6.2642, 31.4021) -> (6.194, 31.3397) construction
  line L926 (6.194, 31.3397) -> (6.0849, 31.3397) construction
  spline S231 degree 2 poles (6.0849, 31.3397) (5.9836, 31.3397) (5.8355, 31.4644) (5.8355, 31.5891) knots 0 0 0 1 2 2 2
  line L927 (6.0849, 31.3397) -> (5.9836, 31.3397) construction
  line L928 (5.9836, 31.3397) -> (5.8355, 31.4644) construction
  line L929 (5.8355, 31.4644) -> (5.8355, 31.5891) construction
  line L930 (5.8355, 31.5891) -> (5.8355, 34.5821)
  spline S232 degree 2 poles (5.8355, 34.5821) (5.8355, 34.6834) (5.9095, 34.7692) knots 0 0 0 1 1 1
  line L931 (5.8355, 34.5821) -> (5.8355, 34.6834) construction
  line L932 (5.8355, 34.6834) -> (5.9095, 34.7692) construction
  spline S233 degree 2 poles (5.9095, 34.7692) (5.9836, 34.8315) (6.0849, 34.8315) knots 0 0 0 1 1 1
  line L933 (5.9095, 34.7692) -> (5.9836, 34.8315) construction
  line L934 (5.9836, 34.8315) -> (6.0849, 34.8315) construction
  spline S234 degree 2 poles (6.0849, 34.8315) (6.1823, 34.8315) (6.3343, 34.7068) (6.3343, 34.5821) knots 0 0 0 1 2 2 2
  line L935 (6.0849, 34.8315) -> (6.1823, 34.8315) construction
  line L936 (6.1823, 34.8315) -> (6.3343, 34.7068) construction
  line L937 (6.3343, 34.7068) -> (6.3343, 34.5821) construction
  spline S235 degree 2 poles (2.8425, 32.3374) (2.8425, 32.1269) (2.9867, 31.9827) knots 0 0 0 1 1 1
  line L938 (2.8425, 32.3374) -> (2.8425, 32.1269) construction
  line L939 (2.8425, 32.1269) -> (2.9867, 31.9827) construction
  spline S236 degree 2 poles (2.9867, 31.9827) (3.0607, 31.9165) (3.1465, 31.8736) knots 0 0 0 1 1 1
  line L940 (2.9867, 31.9827) -> (3.0607, 31.9165) construction
  line L941 (3.0607, 31.9165) -> (3.1465, 31.8736) construction
  spline S237 degree 2 poles (3.1465, 31.8736) (3.2517, 31.8385) (3.3413, 31.8385) knots 0 0 0 1 1 1
  line L942 (3.1465, 31.8736) -> (3.2517, 31.8385) construction
  line L943 (3.2517, 31.8385) -> (3.3413, 31.8385) construction
  line L944 (3.3413, 31.8385) -> (4.5884, 31.8385)
  spline S238 degree 2 poles (4.5884, 31.8385) (4.6936, 31.8385) (4.8378, 31.6866) (4.8378, 31.5891) knots 0 0 0 1 2 2 2
  line L945 (4.5884, 31.8385) -> (4.6936, 31.8385) construction
  line L946 (4.6936, 31.8385) -> (4.8378, 31.6866) construction
  line L947 (4.8378, 31.6866) -> (4.8378, 31.5891) construction
  spline S239 degree 2 poles (4.8378, 31.5891) (4.8378, 31.5034) (4.7131, 31.3397) (4.5884, 31.3397) knots 0 0 0 1 2 2 2
  line L948 (4.8378, 31.5891) -> (4.8378, 31.5034) construction
  line L949 (4.8378, 31.5034) -> (4.7131, 31.3397) construction
  line L950 (4.7131, 31.3397) -> (4.5884, 31.3397) construction
  line L951 (4.5884, 31.3397) -> (3.3413, 31.3397)
  spline S240 degree 2 poles (3.3413, 31.3397) (2.936, 31.3397) (2.3437, 31.9204) (2.3437, 32.3374) knots 0 0 0 1 2 2 2
  line L952 (3.3413, 31.3397) -> (2.936, 31.3397) construction
  line L953 (2.936, 31.3397) -> (2.3437, 31.9204) construction
  line L954 (2.3437, 31.9204) -> (2.3437, 32.3374) construction
  line L955 (2.3437, 32.3374) -> (2.3437, 33.8339)
  spline S241 degree 2 poles (2.3437, 33.8339) (2.3437, 34.2353) (2.9204, 34.8315) (3.3413, 34.8315) knots 0 0 0 1 2 2 2
  line L956 (2.3437, 33.8339) -> (2.3437, 34.2353) construction
  line L957 (2.3437, 34.2353) -> (2.9204, 34.8315) construction
  line L958 (2.9204, 34.8315) -> (3.3413, 34.8315) construction
  line L959 (3.3413, 34.8315) -> (3.8401, 34.8315)
  spline S242 degree 2 poles (3.8401, 34.8315) (4.2454, 34.8315) (4.8378, 34.2509) (4.8378, 33.8339) knots 0 0 0 1 2 2 2
  line L960 (3.8401, 34.8315) -> (4.2454, 34.8315) construction
  line L961 (4.2454, 34.8315) -> (4.8378, 34.2509) construction
  line L962 (4.8378, 34.2509) -> (4.8378, 33.8339) construction
  line L963 (4.8378, 33.8339) -> (4.8378, 33.0856)
  spline S243 degree 2 poles (4.8378, 33.0856) (4.8378, 32.8362) (4.5884, 32.8362) knots 0 0 0 1 1 1
  line L964 (4.8378, 33.0856) -> (4.8378, 32.8362) construction
  line L965 (4.8378, 32.8362) -> (4.5884, 32.8362) construction
  spline S244 degree 2 poles (-5.6376, 31.5891) (-5.6376, 31.4722) (-5.7078, 31.4021) knots 0 0 0 1 1 1
  line L966 (-5.6376, 31.5891) -> (-5.6376, 31.4722) construction
  line L967 (-5.6376, 31.4722) -> (-5.7078, 31.4021) construction
  spline S245 degree 2 poles (-5.7078, 31.4021) (-5.7779, 31.3397) (-5.8871, 31.3397) knots 0 0 0 1 1 1
  line L968 (-5.7078, 31.4021) -> (-5.7779, 31.3397) construction
  line L969 (-5.7779, 31.3397) -> (-5.8871, 31.3397) construction
  spline S246 degree 2 poles (-5.8871, 31.3397) (-5.9884, 31.3397) (-6.1365, 31.4644) (-6.1365, 31.5891) knots 0 0 0 1 2 2 2
  line L970 (-5.8871, 31.3397) -> (-5.9884, 31.3397) construction
  line L971 (-5.9884, 31.3397) -> (-6.1365, 31.4644) construction
  line L972 (-6.1365, 31.4644) -> (-6.1365, 31.5891) construction
  line L973 (-6.1365, 31.5891) -> (-6.1365, 34.5821)
  spline S247 degree 2 poles (-6.1365, 34.5821) (-6.1365, 34.8315) (-5.8871, 34.8315) knots 0 0 0 1 1 1
  line L974 (-6.1365, 34.5821) -> (-6.1365, 34.8315) construction
  line L975 (-6.1365, 34.8315) -> (-5.8871, 34.8315) construction
  line L976 (-5.8871, 34.8315) -> (-3.6423, 34.8315)
  spline S248 degree 2 poles (-3.6423, 34.8315) (-3.237, 34.8315) (-2.6447, 34.2509) (-2.6447, 33.8339) knots 0 0 0 1 2 2 2
  line L977 (-3.6423, 34.8315) -> (-3.237, 34.8315) construction
  line L978 (-3.237, 34.8315) -> (-2.6447, 34.2509) construction
  line L979 (-2.6447, 34.2509) -> (-2.6447, 33.8339) construction
  line L980 (-2.6447, 33.8339) -> (-2.6447, 31.5891)
  spline S249 degree 2 poles (-2.6447, 31.5891) (-2.6447, 31.4722) (-2.7148, 31.4021) knots 0 0 0 1 1 1
  line L981 (-2.6447, 31.5891) -> (-2.6447, 31.4722) construction
  line L982 (-2.6447, 31.4722) -> (-2.7148, 31.4021) construction
  spline S250 degree 2 poles (-2.7148, 31.4021) (-2.785, 31.3397) (-2.8941, 31.3397) knots 0 0 0 1 1 1
  line L983 (-2.7148, 31.4021) -> (-2.785, 31.3397) construction
  line L984 (-2.785, 31.3397) -> (-2.8941, 31.3397) construction
  spline S251 degree 2 poles (-2.8941, 31.3397) (-2.9954, 31.3397) (-3.1435, 31.4644) (-3.1435, 31.5891) knots 0 0 0 1 2 2 2
  line L985 (-2.8941, 31.3397) -> (-2.9954, 31.3397) construction
  line L986 (-2.9954, 31.3397) -> (-3.1435, 31.4644) construction
  line L987 (-3.1435, 31.4644) -> (-3.1435, 31.5891) construction
  line L988 (-3.1435, 31.5891) -> (-3.1435, 33.8339)
  spline S252 degree 2 poles (-3.1435, 33.8339) (-3.1435, 34.0443) (-3.4241, 34.3327) (-3.6423, 34.3327) knots 0 0 0 1 2 2 2
  line L989 (-3.1435, 33.8339) -> (-3.1435, 34.0443) construction
  line L990 (-3.1435, 34.0443) -> (-3.4241, 34.3327) construction
  line L991 (-3.4241, 34.3327) -> (-3.6423, 34.3327) construction
  spline S253 degree 2 poles (-4.1411, 31.5891) (-4.1411, 31.4722) (-4.2113, 31.4021) knots 0 0 0 1 1 1
  line L992 (-4.1411, 31.5891) -> (-4.1411, 31.4722) construction
  line L993 (-4.1411, 31.4722) -> (-4.2113, 31.4021) construction
  spline S254 degree 2 poles (-4.2113, 31.4021) (-4.2814, 31.3397) (-4.3906, 31.3397) knots 0 0 0 1 1 1
  line L994 (-4.2113, 31.4021) -> (-4.2814, 31.3397) construction
  line L995 (-4.2814, 31.3397) -> (-4.3906, 31.3397) construction
  spline S255 degree 2 poles (-4.3906, 31.3397) (-4.4919, 31.3397) (-4.64, 31.4644) (-4.64, 31.5891) knots 0 0 0 1 2 2 2
  line L996 (-4.3906, 31.3397) -> (-4.4919, 31.3397) construction
  line L997 (-4.4919, 31.3397) -> (-4.64, 31.4644) construction
  line L998 (-4.64, 31.4644) -> (-4.64, 31.5891) construction
  line L999 (-8.2331, 31.3397) -> (-8.5293, 31.3397)
  spline S256 degree 2 poles (-8.5293, 31.3397) (-8.9775, 31.3397) (-9.6283, 31.9749) (-9.6283, 32.4387) knots 0 0 0 1 2 2 2
  line L1000 (-8.5293, 31.3397) -> (-8.9775, 31.3397) construction
  line L1001 (-8.9775, 31.3397) -> (-9.6283, 31.9749) construction
  line L1002 (-9.6283, 31.9749) -> (-9.6283, 32.4387) construction
  line L1003 (-9.6283, 32.4387) -> (-9.6283, 33.7325)
  spline S257 degree 2 poles (-9.6283, 33.7325) (-9.6283, 34.1729) (-8.9853, 34.8315) (-8.5293, 34.8315) knots 0 0 0 1 2 2 2
  line L1004 (-9.6283, 33.7325) -> (-9.6283, 34.1729) construction
  line L1005 (-9.6283, 34.1729) -> (-8.9853, 34.8315) construction
  line L1006 (-8.9853, 34.8315) -> (-8.5293, 34.8315) construction
  line L1007 (-8.5293, 34.8315) -> (-8.2331, 34.8315)
  spline S258 degree 2 poles (-8.2331, 34.8315) (-7.785, 34.8315) (-7.1341, 34.1924) (-7.1341, 33.7325) knots 0 0 0 1 2 2 2
  line L1008 (-8.2331, 34.8315) -> (-7.785, 34.8315) construction
  line L1009 (-7.785, 34.8315) -> (-7.1341, 34.1924) construction
  line L1010 (-7.1341, 34.1924) -> (-7.1341, 33.7325) construction
  line L1011 (-7.1341, 33.7325) -> (-7.1341, 32.4387)
  spline S259 degree 2 poles (-7.1341, 32.4387) (-7.1341, 31.9905) (-7.7733, 31.3397) (-8.2331, 31.3397) knots 0 0 0 1 2 2 2
  line L1012 (-7.1341, 32.4387) -> (-7.1341, 31.9905) construction
  line L1013 (-7.1341, 31.9905) -> (-7.7733, 31.3397) construction
  line L1014 (-7.7733, 31.3397) -> (-8.2331, 31.3397) construction
  spline S260 degree 2 poles (0.7423, 63.1472) (0.6722, 63.0848) (0.5631, 63.0848) knots 0 0 0 1 1 1
  line L1015 (0.7423, 63.1472) -> (0.6722, 63.0848) construction
  line L1016 (0.6722, 63.0848) -> (0.5631, 63.0848) construction
  spline S261 degree 2 poles (0.5631, 63.0848) (0.4617, 63.0848) (0.3136, 63.2095) (0.3136, 63.3342) knots 0 0 0 1 2 2 2
  line L1017 (0.5631, 63.0848) -> (0.4617, 63.0848) construction
  line L1018 (0.4617, 63.0848) -> (0.3136, 63.2095) construction
  line L1019 (0.3136, 63.2095) -> (0.3136, 63.3342) construction
  spline S262 degree 2 poles (-1.1945, 63.2563) (-1.2218, 63.1745) (-1.2881, 63.1238) knots 0 0 0 1 1 1
  line L1020 (-1.1945, 63.2563) -> (-1.2218, 63.1745) construction
  line L1021 (-1.2218, 63.1745) -> (-1.2881, 63.1238) construction
  spline S263 degree 2 poles (-1.2881, 63.1238) (-1.3037, 63.1121) (-1.4206, 63.0848) knots 0 0 0 1 1 1
  line L1022 (-1.2881, 63.1238) -> (-1.3037, 63.1121) construction
  line L1023 (-1.3037, 63.1121) -> (-1.4206, 63.0848) construction
  spline S264 degree 2 poles (-1.4206, 63.0848) (-1.5219, 63.0848) (-1.5959, 63.155) knots 0 0 0 1 1 1
  line L1024 (-1.4206, 63.0848) -> (-1.5219, 63.0848) construction
  line L1025 (-1.5219, 63.0848) -> (-1.5959, 63.155) construction
  spline S265 degree 2 poles (-1.5959, 63.155) (-1.6778, 63.2212) (-1.6778, 63.3225) knots 0 0 0 1 1 1
  line L1026 (-1.5959, 63.155) -> (-1.6778, 63.2212) construction
  line L1027 (-1.6778, 63.2212) -> (-1.6778, 63.3225) construction
  spline S266 degree 2 poles (-0.6723, 66.4052) (-0.6217, 66.5766) (-0.4385, 66.5766) knots 0 0 0 1 1 1
  line L1028 (-0.6723, 66.4052) -> (-0.6217, 66.5766) construction
  line L1029 (-0.6217, 66.5766) -> (-0.4385, 66.5766) construction
  line L1030 (-0.4385, 66.5766) -> (0.5631, 66.5766)
  spline S267 degree 2 poles (0.5631, 66.5766) (0.8125, 66.5766) (0.8125, 66.3272) knots 0 0 0 1 1 1
  line L1031 (0.5631, 66.5766) -> (0.8125, 66.5766) construction
  line L1032 (0.8125, 66.5766) -> (0.8125, 66.3272) construction
  line L1033 (0.8125, 66.3272) -> (0.8125, 63.3342)
  spline S268 degree 2 poles (0.8125, 63.3342) (0.8125, 63.2173) (0.7423, 63.1472) knots 0 0 0 1 1 1
  line L1034 (0.8125, 63.3342) -> (0.8125, 63.2173) construction
  line L1035 (0.8125, 63.2173) -> (0.7423, 63.1472) construction
  line L1036 (-3.7783, 63.0848) -> (-4.0745, 63.0848)
  spline S269 degree 2 poles (-4.0745, 63.0848) (-4.5227, 63.0848) (-5.1735, 63.72) (-5.1735, 64.1838) knots 0 0 0 1 2 2 2
  line L1037 (-4.0745, 63.0848) -> (-4.5227, 63.0848) construction
  line L1038 (-4.5227, 63.0848) -> (-5.1735, 63.72) construction
  line L1039 (-5.1735, 63.72) -> (-5.1735, 64.1838) construction
  line L1040 (-5.1735, 64.1838) -> (-5.1735, 65.4776)
  spline S270 degree 2 poles (-5.1735, 65.4776) (-5.1735, 65.918) (-4.5305, 66.5766) (-4.0745, 66.5766) knots 0 0 0 1 2 2 2
  line L1041 (-5.1735, 65.4776) -> (-5.1735, 65.918) construction
  line L1042 (-5.1735, 65.918) -> (-4.5305, 66.5766) construction
  line L1043 (-4.5305, 66.5766) -> (-4.0745, 66.5766) construction
  line L1044 (-4.0745, 66.5766) -> (-3.7783, 66.5766)
  spline S271 degree 2 poles (-3.7783, 66.5766) (-3.3302, 66.5766) (-2.6793, 65.9375) (-2.6793, 65.4776) knots 0 0 0 1 2 2 2
  line L1045 (-3.7783, 66.5766) -> (-3.3302, 66.5766) construction
  line L1046 (-3.3302, 66.5766) -> (-2.6793, 65.9375) construction
  line L1047 (-2.6793, 65.9375) -> (-2.6793, 65.4776) construction
  line L1048 (-2.6793, 65.4776) -> (-2.6793, 64.1838)
  spline S272 degree 2 poles (-2.6793, 64.1838) (-2.6793, 63.7356) (-3.3185, 63.0848) (-3.7783, 63.0848) knots 0 0 0 1 2 2 2
  line L1049 (-2.6793, 64.1838) -> (-2.6793, 63.7356) construction
  line L1050 (-2.6793, 63.7356) -> (-3.3185, 63.0848) construction
  line L1051 (-3.3185, 63.0848) -> (-3.7783, 63.0848) construction
  spline S273 degree 2 poles (-6.2413, 63.1472) (-6.3115, 63.0848) (-6.4206, 63.0848) knots 0 0 0 1 1 1
  line L1052 (-6.2413, 63.1472) -> (-6.3115, 63.0848) construction
  line L1053 (-6.3115, 63.0848) -> (-6.4206, 63.0848) construction
  spline S274 degree 2 poles (-6.4206, 63.0848) (-6.5219, 63.0848) (-6.67, 63.2095) (-6.67, 63.3342) knots 0 0 0 1 2 2 2
  line L1054 (-6.4206, 63.0848) -> (-6.5219, 63.0848) construction
  line L1055 (-6.5219, 63.0848) -> (-6.67, 63.2095) construction
  line L1056 (-6.67, 63.2095) -> (-6.67, 63.3342) construction
  line L1057 (-6.67, 63.3342) -> (-6.67, 65.579)
  spline S275 degree 2 poles (-6.67, 65.579) (-6.67, 65.7894) (-6.9506, 66.0778) (-7.1688, 66.0778) knots 0 0 0 1 2 2 2